Autodesk Fusion 360 part; units mm, degrees
(part 7 of 11)
  arc A26 (6.6572, -81.7997) -> (6.7986, -81.4582) centre (6.6572, -81.5997) ccw
  line L277 (19.9198, -134.2989) -> (19.8859, -134.2627)
  line L278 (4.42, -81.7997) -> (6.6572, -81.7997)
  line L279 (4.62, -81.9997) -> (6.6572, -81.9997)
  line L280 (20.0926, -134.6222) -> (20.0773, -134.5717)
  line L281 (19.9148, -134.7519) -> (19.9083, -134.7127)
  line L282 (4.42, -81.7997) -> (6.6572, -81.7997)
  arc A27 (6.6572, -81.7997) -> (6.7986, -81.4582) centre (6.6572, -81.5997) ccw
  line L283 (20.1046, -134.6736) -> (20.0926, -134.6222)
  line L284 (1.92, -84.6997) -> (3.2765, -84.6997)
  arc A28 (6.6572, -81.9997) -> (6.94, -81.3168) centre (6.6572, -81.5997) ccw
  line L285 (20.12, -134.8278) -> (20.1184, -134.7783)
  line L286 (4.42, -83.439) -> (4.42, -81.7997)
  line L287 (19.8993, -134.674) -> (19.8878, -134.636)
  line L288 (1.72, -84.4997) -> (3.3593, -84.4997)
  line L289 (20.012, -134.4275) -> (19.9841, -134.3827)
  line L290 (4.42, -83.439) -> (4.42, -81.7997)
  line L291 (19.9083, -134.7127) -> (19.8993, -134.674)
  line L292 (1.72, -84.4997) -> (3.3593, -84.4997)
  line L293 (-3, -220) -> (20, -220)
  line L294 (19.9148, -134.7519) -> (19.9083, -134.7127)
  line L295 (19.9841, -134.3827) -> (19.9533, -134.3397)
  line L296 (19.8878, -134.636) -> (19.8738, -134.5988)
  line L297 (-0.08, -85.0997) -> (-0.0787, -85.2079)
  line L298 (20.0587, -134.5222) -> (20.0369, -134.4741)
  line L299 (-0.28, -81.4997) -> (-0.28, -85.1009)
  line L300 (19.92, -134.8311) -> (19.9187, -134.7914)
  line L301 (-0.08, -85.0997) -> (-0.0787, -85.2079)
  line L302 (19.9187, -134.7914) -> (19.9148, -134.7519)
  line L303 (19.8387, -134.5276) -> (19.8177, -134.4938)
  line L304 (-0.28, -85.1009) -> (-0.2786, -85.2189)
  line L305 (-0.0787, -85.2079) -> (-0.0748, -85.2474)
  line L306 (-0.2786, -85.2189) -> (-0.2732, -85.2736)
  line L307 (20.1132, -134.7258) -> (20.1046, -134.6736)
  line L308 (20.0773, -134.5717) -> (20.0587, -134.5222)
  line L309 (19.8993, -134.674) -> (19.8878, -134.636)
  line L310 (19.9533, -134.3397) -> (19.9198, -134.2989)
  line L311 (20.1184, -134.7783) -> (20.1132, -134.7258)
  line L312 (18.12, -57.2997) -> (18.12, -62.6997)
  line L313 (-0.0787, -85.2079) -> (-0.0748, -85.2474)
  line L314 (-0.0748, -85.2474) -> (-0.0683, -85.2866)
  line L315 (19.8574, -134.5626) -> (19.8387, -134.5276)
  line L316 (-0.08, -81.4997) -> (-0.08, -85.0997)
  line L317 (-0.0683, -85.2866) -> (-0.0593, -85.3253)
  line L318 (19.7946, -134.4616) -> (19.7694, -134.4308)
  line L319 (7.0807, -86.0997) -> (4.42, -83.439)
  line L320 (3.3593, -84.4997) -> (6.02, -87.1603)
  line L321 (19.7946, -134.4616) -> (19.7694, -134.4308)
  line L322 (-0.2732, -85.2736) -> (-0.2646, -85.3257)
  line L323 (1.72, -86.7368) -> (1.72, -84.4997)
  line L324 (-0.08, -81.4997) -> (-0.08, -85.0997)
  line L325 (19.9083, -134.7127) -> (19.8993, -134.674)
  line L326 (19.8177, -134.4938) -> (19.7946, -134.4616)
  line L327 (19.8177, -134.4938) -> (19.7946, -134.4616)
  line L328 (-0.0748, -85.2474) -> (-0.0683, -85.2866)
  line L329 (19.9187, -134.7914) -> (19.9148, -134.7519)
  line L330 (7.1635, -85.8997) -> (4.62, -83.3562)
  line L331 (19.8738, -134.5988) -> (19.8574, -134.5626)
  line L332 (1.92, -86.7368) -> (1.92, -84.6997)
  line L333 (7.0807, -86.0997) -> (4.42, -83.439)
  line L334 (19.92, -134.8311) -> (19.9187, -134.7914)
  line L335 (19.8878, -134.636) -> (19.8738, -134.5988)
  line L336 (20.0369, -134.4741) -> (20.012, -134.4275)
  line L337 (-0.0683, -85.2866) -> (-0.0593, -85.3253)
  line L338 (19.8387, -134.5276) -> (19.8177, -134.4938)
  line L339 (1.72, -86.7368) -> (1.72, -84.4997)
  line L340 (19.8574, -134.5626) -> (19.8387, -134.5276)
  line L341 (3.3593, -84.4997) -> (6.02, -87.1603)
  line L342 (3.2765, -84.6997) -> (5.82, -87.2432)
  line L343 (9.7959, -85.8997) -> (7.1635, -85.8997)
  circle A29 centre (9.92, -89.9997) radius 2.1
  arc A30 (18.6028, -132.9797) -> (17.92, -133.2625) centre (18.32, -133.2625) ccw
  line L344 (19.8993, -154.674) -> (19.8878, -154.636)
  line L345 (19.8574, -154.5626) -> (19.8387, -154.5276)
  line L346 (20.1046, -154.6736) -> (20.0926, -154.6222)
  line L347 (19.7946, -154.4616) -> (19.7694, -154.4308)
  line L348 (20.0369, -154.4741) -> (20.012, -154.4275)
  line L349 (19.9083, -154.7127) -> (19.8993, -154.674)
  line L350 (19.8738, -154.5988) -> (19.8574, -154.5626)
  line L351 (19.7694, -154.4308) -> (19.7422, -154.4019)
  line L352 (20.0773, -154.5717) -> (20.0587, -154.5222)
  line L353 (7.0807, -6.0997) -> (4.42, -3.439)
  line L354 (1.72, -4.4997) -> (3.3593, -4.4997)
  line L355 (19.92, -1.4997) -> (19.92, -0.4997)
  line L356 (-0.0787, -5.2079) -> (-0.0748, -5.2474)
  line L357 (18.42, 0.0003) -> (14.7514, 0.0003)
  arc A31 (19.92, -0.4997) -> (19.42, 0.0003) centre (19.42, -0.4997) ccw
  line L358 (3.3593, -4.4997) -> (6.02, -7.1603)
  line L359 (19.92, -1.4997) -> (19.92, -0.4997)
  line L360 (19.7946, -14.4616) -> (19.7694, -14.4308)
  line L361 (-0.0459, -5.7366) -> (1.2372, -7.0197)
  line L362 (9.713, -26.0997) -> (7.0807, -26.0997)
  line L363 (9.713, -26.0997) -> (7.0807, -26.0997)
  line L364 (19.9841, -14.3827) -> (19.9533, -14.3397)
  line L365 (19.9083, -45.2866) -> (19.9148, -45.2474)
  line L366 (-0.0683, -5.2866) -> (-0.0593, -5.3253)
  line L367 (10.127, -13.8997) -> (12.7593, -13.8997)
  line L368 (19.9533, -14.3397) -> (19.9198, -14.2989)
  line L369 (19.7694, -14.4308) -> (19.7422, -14.4019)
  line L370 (20.12, -1.4997) -> (20.12, -0.4997)
  line L371 (19.8177, -14.4938) -> (19.7946, -14.4616)
  line L372 (7.0807, -6.0997) -> (4.42, -3.439)
  line L373 (19.92, -14.8997) -> (19.9187, -14.7914)
  line L374 (19.8993, -14.674) -> (19.8878, -14.636)
  line L375 (4.62, -1.9997) -> (6.6572, -1.9997)
  arc A32 (1.2372, -27.0197) -> (1.92, -26.7368) centre (1.52, -26.7368) ccw
  line L376 (19.9148, -14.7519) -> (19.9083, -14.7127)
  line L377 (19.42, 0.2003) -> (18.42, 0.2003)
  line L378 (0.0978, -5.5975) -> (1.3786, -6.8782)
  line L379 (18.42, 0.2003) -> (14.7482, 0.2003)
  line L380 (1.72, -4.4997) -> (3.3593, -4.4997)
  line L381 (19.42, 0.0003) -> (18.42, 0.0003)
  line L382 (7.1635, -5.8997) -> (4.62, -3.3562)
  line L383 (-0.0748, -5.2474) -> (-0.0683, -5.2866)
  line L384 (19.7946, -45.5378) -> (19.8177, -45.5055)
  line L385 (19.8738, -45.4005) -> (19.8878, -45.3633)
  line L386 (9.92, -26.3066) -> (9.713, -26.0997)
  line L387 (9.7959, -14.0997) -> (9.92, -13.9755)
  arc A33 (19.92, -0.4997) -> (19.42, 0.0003) centre (19.42, -0.4997) ccw
  line L388 (3.2765, -4.6997) -> (5.82, -7.2432)
  line L389 (19.42, 0.0003) -> (18.42, 0.0003)
  line L390 (19.8177, -14.4938) -> (19.7946, -14.4616)
  line L391 (12.7593, -26.0997) -> (10.127, -26.0997)
  line L392 (7.0807, -13.8997) -> (9.713, -13.8997)
  line L393 (1.92, -6.7368) -> (1.92, -4.6997)
  line L394 (-0.28, -5.1009) -> (-0.2786, -5.2189)
  line L395 (20.1046, -14.6736) -> (20.0926, -14.6222)
  line L396 (19.8387, -14.5276) -> (19.8177, -14.4938)
  line L397 (20.0773, -14.5717) -> (20.0587, -14.5222)
  arc A34 (6.6572, -1.7997) -> (6.7986, -1.4582) centre (6.6572, -1.5997) ccw
  arc A35 (20.12, -0.4997) -> (19.42, 0.2003) centre (19.42, -0.4997) ccw
  line L398 (1.72, -6.7368) -> (1.72, -4.4997)
  line L399 (10.127, -13.8997) -> (12.7593, -13.8997)
  line L400 (3.3593, -4.4997) -> (6.02, -7.1603)
  line L401 (3.7635, -162.4997) -> (1.92, -162.4997)
  line L402 (1.72, -6.7368) -> (1.72, -4.4997)
  line L403 (18.42, 0.0003) -> (14.7514, 0.0003)
  line L404 (19.8878, -14.636) -> (19.8738, -14.5988)
  arc A36 (1.2372, -167.0197) -> (1.92, -166.7368) centre (1.52, -166.7368) ccw
  line L405 (9.92, -13.6927) -> (10.127, -13.8997)
  line L406 (19.7946, -14.4616) -> (19.7694, -14.4308)
  line L407 (19.9083, -14.7127) -> (19.8993, -14.674)
  line L408 (0.0978, -5.5975) -> (1.3786, -6.8782)
  line L409 (19.92, -14.8997) -> (19.9187, -14.7914)
  line L410 (19.7694, -14.4308) -> (19.7422, -14.4019)
  line L411 (5.4921, 0.0923) -> (5.4455, 0.1172)
  line L412 (0.0978, -25.5975) -> (1.3786, -26.8782)
  line L413 (-0.0593, -25.3253) -> (-0.0478, -25.3633)
  line L414 (19.8574, -14.5626) -> (19.8387, -14.5276)
  line L415 (19.9187, -14.7914) -> (19.9148, -14.7519)
  line L416 (6.7986, -1.4582) -> (5.5178, -0.1775)
  arc A37 (6.6572, -1.7997) -> (6.7986, -1.4582) centre (6.6572, -1.5997) ccw
  line L417 (4.42, -1.7997) -> (6.6572, -1.7997)
  line L418 (20.012, -14.4275) -> (19.9841, -14.3827)
  line L419 (-0.1969, -25.5252) -> (-0.172, -25.5718)
  line L420 (14.6722, -0.0049) -> (14.633, -0.0113)
  line L421 (14.5943, -0.0203) -> (14.5563, -0.0319)
  line L422 (14.3945, 0.1172) -> (14.3479, 0.0923)
  line L423 (5.4581, -0.1251) -> (5.4258, -0.102)
  line L424 (6.7986, -1.4582) -> (5.5178, -0.1775)
  line L425 (19.8878, -14.636) -> (19.8738, -14.5988)
  line L426 (19.8738, -14.5988) -> (19.8574, -14.5626)
  line L427 (19.9083, -14.7127) -> (19.8993, -14.674)
  line L428 (19.9187, -14.7914) -> (19.9148, -14.7519)
  line L429 (5.3974, 0.139) -> (5.348, 0.1576)
  line L430 (20.0587, -14.5222) -> (20.0369, -14.4741)
  arc A38 (1.3786, -26.8782) -> (1.72, -26.7368) centre (1.52, -26.7368) ccw
  line L431 (14.6987, 0.1987) -> (14.6461, 0.1935)
  line L432 (20.1132, -14.7258) -> (20.1046, -14.6736)
  line L433 (14.4142, -0.102) -> (14.3819, -0.1251)
  line L434 (20.12, -14.8985) -> (20.1186, -14.7804)
  line L435 (-0.2732, -25.2736) -> (-0.2646, -25.3257)
  arc A39 (1.3786, -26.8782) -> (1.72, -26.7368) centre (1.52, -26.7368) ccw
  line L436 (14.3512, -0.1503) -> (14.3222, -0.1775)
  line L437 (14.4479, -0.081) -> (14.4142, -0.102)
  line L438 (14.633, -0.0113) -> (14.5943, -0.0203)
  line L439 (5.537, 0.0644) -> (5.4921, 0.0923)
  line L440 (14.594, 0.1849) -> (14.5425, 0.1729)
  line L441 (19.8993, -14.674) -> (19.8878, -14.636)
  line L442 (-0.2786, -25.2189) -> (-0.2732, -25.2736)
  line L443 (5.4258, -0.102) -> (5.3921, -0.081)
  arc A40 (6.6572, -1.9997) -> (6.94, -1.3168) centre (6.6572, -1.5997) ccw
  line L444 (-0.0338, -25.4005) -> (-0.0174, -25.4367)
  line L445 (5.2837, -0.0319) -> (5.2457, -0.0203)
  line L446 (14.3512, -0.1503) -> (14.3222, -0.1775)
  line L447 (5.2457, -0.0203) -> (5.207, -0.0113)
  line L448 (5.2457, -0.0203) -> (5.207, -0.0113)
  line L449 (-0.28, -25.1009) -> (-0.2786, -25.2189)
  line L450 (19.8574, -14.5626) -> (19.8387, -14.5276)
  line L451 (-0.1133, -25.6596) -> (-0.0798, -25.7004)
  line L452 (19.8738, -14.5988) -> (19.8574, -14.5626)
  line L453 (19.8387, -14.5276) -> (19.8177, -14.4938)
  line L454 (0.0978, -25.5975) -> (1.3786, -26.8782)
  line L455 (4.42, -1.7997) -> (6.6572, -1.7997)
  line L456 (19.9198, -14.2989) -> (19.8859, -14.2627)
  line L457 (20.1186, -14.7804) -> (20.1132, -14.7258)
  line L458 (20.0369, -14.4741) -> (20.012, -14.4275)
  arc A41 (18.6028, -12.9797) -> (17.92, -13.2625) centre (18.32, -13.2625) ccw
  line L459 (19.9148, -14.7519) -> (19.9083, -14.7127)
  line L460 (20.0926, -14.6222) -> (20.0773, -14.5717)
  line L461 (-0.0748, -25.2474) -> (-0.0683, -25.2866)
  line L462 (5.2975, 0.1729) -> (5.246, 0.1849)
  line L463 (-0.0748, -25.2474) -> (-0.0683, -25.2866)
  arc A42 (18.4614, -13.1211) -> (18.12, -13.2625) centre (18.32, -13.2625) ccw
  line L464 (-0.0787, -25.2079) -> (-0.0748, -25.2474)
  arc A43 (18.4614, -13.1211) -> (18.12, -13.2625) centre (18.32, -13.2625) ccw
  line L465 (-0.0338, -25.4005) -> (-0.0174, -25.4367)
  line L466 (14.3819, -0.1251) -> (14.3512, -0.1503)
  line L467 (18.12, -13.2625) -> (18.12, -15.4997)
  line L468 (14.633, -0.0113) -> (14.5943, -0.0203)
  line L469 (5.2837, -0.0319) -> (5.2457, -0.0203)
  line L470 (-0.0174, -25.4367) -> (0.0013, -25.4717)
  line L471 (17.92, -13.2625) -> (17.92, -15.2997)
  line L472 (14.6461, 0.1935) -> (14.594, 0.1849)
  line L473 (-0.0787, -25.2079) -> (-0.0748, -25.2474)
  line L474 (5.4258, -0.102) -> (5.3921, -0.081)
  line L475 (5.246, 0.1849) -> (5.1939, 0.1935)
  line L476 (0.0223, -25.5055) -> (0.0454, -25.5378)
  line L477 (14.3479, 0.0923) -> (14.303, 0.0644)
  line L478 (-0.1441, -25.6166) -> (-0.1133, -25.6596)
  line L479 (6.02, -12.839) -> (3.3593, -15.4997)
  line L480 (5.348, 0.1576) -> (5.2975, 0.1729)
  line L481 (16.4807, -15.4997) -> (13.82, -12.839)
  line L482 (0.0013, -25.4717) -> (0.0223, -25.5055)
  line L483 (14.4479, -0.081) -> (14.4142, -0.102)
  line L484 (5.1283, -0.001) -> (5.0886, 0.0003)
  line L485 (-0.08, -25.0997) -> (-0.0787, -25.2079)
  line L486 (-0.0174, -25.4367) -> (0.0013, -25.4717)
  line L487 (19.92, -25.0997) -> (19.92, -14.8997)
  line L488 (5.1283, -0.001) -> (5.0886, 0.0003)
  line L489 (-0.08, -25.0997) -> (-0.0787, -25.2079)
  line L490 (5.1413, 0.1987) -> (5.0918, 0.2003)
  line L491 (-0.2526, -25.3771) -> (-0.2373, -25.4277)
  line L492 (18.12, -13.2625) -> (18.12, -15.4997)
  line L493 (5.207, -0.0113) -> (5.1678, -0.0049)
  line L494 (5.3921, -0.081) -> (5.357, -0.0623)
  line L495 (14.483, -0.0623) -> (14.4479, -0.081)
  line L496 (19.7422, -14.4019) -> (18.4614, -13.1211)
  line L497 (16.5635, -15.2997) -> (14.02, -12.7562)
  line L498 (5.357, -0.0623) -> (5.3209, -0.0459)
  line L499 (14.5191, -0.0459) -> (14.483, -0.0623)
  line L500 (17.92, -15.2997) -> (16.5635, -15.2997)
  line L501 (5.3209, -0.0459) -> (5.2837, -0.0319)
  line L502 (-0.0683, -25.2866) -> (-0.0593, -25.3253)
  line L503 (0.0454, -25.5378) -> (0.0706, -25.5685)
  line L504 (-0.0683, -25.2866) -> (-0.0593, -25.3253)
  line L505 (-0.172, -25.5718) -> (-0.1441, -25.6166)
  line L506 (14.7117, -0.001) -> (14.6722, -0.0049)
  line L507 (0.0454, -25.5378) -> (0.0706, -25.5685)
  line L508 (18.12, -15.4997) -> (16.4807, -15.4997)
  line L509 (5.5799, 0.0337) -> (5.537, 0.0644)
  line L510 (19.7422, -14.4019) -> (18.4614, -13.1211)
  line L511 (0.0013, -25.4717) -> (0.0223, -25.5055)
  line L512 (5.1678, -0.0049) -> (5.1283, -0.001)
  line L513 (14.5563, -0.0319) -> (14.5191, -0.0459)
  line L514 (5.6207, 0.0001) -> (5.5799, 0.0337)
  line L515 (19.8859, -14.2627) -> (18.6028, -12.9797)
  line L516 (-0.2373, -25.4277) -> (-0.2187, -25.4771)
  line L517 (-0.0798, -25.7004) -> (-0.0459, -25.7366)
  line L518 (16.4807, -15.4997) -> (13.82, -12.839)
  line L519 (-0.0593, -25.3253) -> (-0.0478, -25.3633)
  line L520 (5.6569, -0.0337) -> (5.6207, 0.0001)
  line L521 (18.12, -15.4997) -> (16.4807, -15.4997)
  line L522 (5.1678, -0.0049) -> (5.1283, -0.001)
  line L523 (-0.0478, -25.3633) -> (-0.0338, -25.4005)
  line L524 (5.4888, -0.1503) -> (5.4581, -0.1251)
  line L525 (20.12, -25.1009) -> (20.12, -14.8985)
  line L526 (14.303, 0.0644) -> (14.2601, 0.0337)
  line L527 (-0.0478, -25.3633) -> (-0.0338, -25.4005)
  line L528 (5.4888, -0.1503) -> (5.4581, -0.1251)
  line L529 (14.5425, 0.1729) -> (14.492, 0.1576)
  line L530 (19.92, -25.0997) -> (19.92, -14.8997)
  line L531 (4.42, -3.439) -> (4.42, -1.7997)
  line L532 (3.3593, -24.4997) -> (6.02, -27.1603)
  line L533 (-0.0459, -25.7366) -> (1.2372, -27.0197)
  line L534 (14.5191, -0.0459) -> (14.483, -0.0623)
  line L535 (-0.08, -0.4997) -> (-0.08, -1.4997)
  line L536 (14.2601, 0.0337) -> (14.2193, 0.0001)
  line L537 (0.0706, -25.5685) -> (0.0978, -25.5975)
  line L538 (14.492, 0.1576) -> (14.4426, 0.139)
  line L539 (6.94, -1.3168) -> (5.6569, -0.0337)
  line L540 (1.72, -17.2997) -> (3.6807, -17.2997)
  line L541 (5.4581, -0.1251) -> (5.4258, -0.102)
  line L542 (19.92, -5.1682) -> (19.92, -1.4997)
  line L543 (7.0807, -46.0997) -> (3.6807, -42.6997)
  line L544 (3.6807, -22.6997) -> (1.72, -22.6997)
  line L545 (5.1939, 0.1935) -> (5.1413, 0.1987)
  line L546 (14.483, -0.0623) -> (14.4479, -0.081)
  line L547 (5.3209, -0.0459) -> (5.2837, -0.0319)
  line L548 (5.207, -0.0113) -> (5.1678, -0.0049)
  line L549 (5.5178, -0.1775) -> (5.4888, -0.1503)
  line L550 (13.82, -7.1603) -> (16.4807, -4.4997)
  line L551 (14.5563, -0.0319) -> (14.5191, -0.0459)
  line L552 (-0.2187, -25.4771) -> (-0.1969, -25.5252)
  line L553 (1.92, -17.4997) -> (3.7635, -17.4997)
  line L554 (0.0223, -25.5055) -> (0.0454, -25.5378)
  line L555 (1.72, -22.6997) -> (1.72, -17.2997)
  line L556 (7.0807, -26.0997) -> (3.6807, -22.6997)
  line L557 (14.6722, -0.0049) -> (14.633, -0.0113)
  line L558 (14.5943, -0.0203) -> (14.5563, -0.0319)
  line L559 (13.82, -192.839) -> (13.82, -190.1995)
  line L560 (15.42, -3.439) -> (12.7593, -6.0997)
  line L561 (5.4455, 0.1172) -> (5.3974, 0.139)
  line L562 (19.92, -45.0997) -> (19.92, -34.8997)
  line L563 (1.72, -22.6997) -> (1.72, -17.2997)
  line L564 (5.3921, -0.081) -> (5.357, -0.0623)
  line L565 (3.7635, -22.4997) -> (1.92, -22.4997)
  line L566 (3.2765, -24.6997) -> (5.82, -27.2432)
  line L567 (14.7514, 0.0003) -> (14.7117, -0.001)
  line L568 (5.5178, -0.1775) -> (5.4888, -0.1503)
  line L569 (16.1593, -42.6997) -> (12.7593, -46.0997)
  line L570 (1.92, -24.6997) -> (3.2765, -24.6997)
  line L571 (13.1828, -1.7997) -> (15.42, -1.7997)
  line L572 (3.6807, -22.6997) -> (1.72, -22.6997)
  arc A44 (0.42, 0.2003) -> (-0.28, -0.4997) centre (0.42, -0.4997) ccw
  line L573 (14.3819, -0.1251) -> (14.3512, -0.1503)
  line L574 (14.4142, -0.102) -> (14.3819, -0.1251)
  line L575 (1.72, -24.4997) -> (3.3593, -24.4997)
  line L576 (20.12, -5.1715) -> (20.12, -1.4997)
  line L577 (13.82, -192.839) -> (13.82, -190.1995)
  arc A45 (0.42, 0.0003) -> (-0.08, -0.4997) centre (0.42, -0.4997) ccw
  line L578 (1.72, -24.4997) -> (3.3593, -24.4997)
  line L579 (15.42, -1.7997) -> (15.42, -3.439)
  line L580 (14.7117, -0.001) -> (14.6722, -0.0049)
  line L581 (14.4426, 0.139) -> (14.3945, 0.1172)
  line L582 (5.357, -0.0623) -> (5.3209, -0.0459)
  line L583 (14.7482, 0.2003) -> (14.6987, 0.1987)
  line L584 (0.0706, -25.5685) -> (0.0978, -25.5975)
  line L585 (14.7514, 0.0003) -> (14.7117, -0.001)
  line L586 (7.1635, -25.8997) -> (3.7635, -22.4997)
  line L587 (-0.2646, -25.3257) -> (-0.2526, -25.3771)
  line L588 (1.92, -22.4997) -> (1.92, -17.4997)
  line L589 (15.22, -1.9997) -> (15.22, -3.3562)
  line L590 (19.92, -5.1682) -> (19.92, -1.4997)
  line L591 (1.72, -17.2997) -> (3.6807, -17.2997)
  line L592 (1.42, 0.0003) -> (0.42, 0.0003)
  line L593 (1.72, -26.7368) -> (1.72, -24.4997)
  line L594 (19.8993, -194.674) -> (19.8878, -194.636)
  line L595 (19.9187, -194.7914) -> (19.9148, -194.7519)
  line L596 (12.7593, -6.0997) -> (10.127, -6.0997)
  line L597 (20.12, -194.8985) -> (20.1186, -194.7804)
  line L598 (1.72, -15.4997) -> (1.72, -13.2625)
  line L599 (13.6201, -9.9997) -> (13.82, -9.7998)
  line L600 (14.02, -10.1167) -> (13.903, -9.9997)
  line L601 (5.0886, 0.0003) -> (1.42, 0.0003)
  line L602 (13.903, -9.9997) -> (14.02, -9.8826)
  line L603 (19.9083, -194.7127) -> (19.8993, -194.674)
  line L604 (19.9148, -34.7519) -> (19.9083, -34.7127)
  line L605 (1.72, -26.7368) -> (1.72, -24.4997)
  arc A46 (1.92, -13.2625) -> (1.2372, -12.9797) centre (1.52, -13.2625) ccw
  line L606 (19.8177, -194.4938) -> (19.7946, -194.4616)
  line L607 (0.0706, -14.4308) -> (0.0454, -14.4616)
  line L608 (19.9187, -34.7914) -> (19.9148, -34.7519)
  line L609 (15.42, -1.7997) -> (15.42, -3.439)
  line L610 (5.0918, 0.2003) -> (1.42, 0.2003)
  line L611 (3.3593, -15.4997) -> (1.72, -15.4997)
  line L612 (7.1635, -45.8997) -> (3.7635, -42.4997)
  line L613 (19.7946, -194.4616) -> (19.7694, -194.4308)
  arc A47 (1.72, -13.2625) -> (1.3786, -13.1211) centre (1.52, -13.2625) ccw
  line L614 (1.3786, -13.1211) -> (0.0978, -14.4019)
  line L615 (19.9841, -194.3827) -> (19.9533, -194.3397)
  line L616 (1.42, 0.2003) -> (0.42, 0.2003)
  line L617 (3.3593, -15.4997) -> (1.72, -15.4997)
  line L618 (19.8177, -194.4938) -> (19.7946, -194.4616)
  line L619 (20.1186, -194.7804) -> (20.1132, -194.7258)
  line L620 (19.8387, -194.5276) -> (19.8177, -194.4938)
  line L621 (19.9148, -194.7519) -> (19.9083, -194.7127)
  arc A48 (13.0414, -1.4582) -> (13.1828, -1.7997) centre (13.1828, -1.5997) ccw
  arc A49 (12.9, -1.3168) -> (13.1828, -1.9997) centre (13.1828, -1.5997) ccw
  line L622 (12.7593, -6.0997) -> (10.127, -6.0997)
  line L623 (1.42, 0.0003) -> (0.42, 0.0003)
  arc A50 (0.42, 0.0003) -> (-0.08, -0.4997) centre (0.42, -0.4997) ccw
  line L624 (1.3786, -13.1211) -> (0.0978, -14.4019)
  line L625 (19.8738, -194.5988) -> (19.8574, -194.5626)
  line L626 (17.92, -37.4997) -> (17.92, -42.4997)
  line L627 (5.0886, 0.0003) -> (1.42, 0.0003)
  circle A51 centre (9.92, -9.9997) radius 2.1
  line L628 (19.9198, -194.2989) -> (19.8859, -194.2627)
  line L629 (19.8387, -194.5276) -> (19.8177, -194.4938)
  line L630 (20.0926, -194.6222) -> (20.0773, -194.5717)
  line L631 (-0.08, -0.4997) -> (-0.08, -1.4997)
  line L632 (-0.28, -0.4997) -> (-0.28, -1.4997)
  line L633 (-0.28, -1.4997) -> (-0.28, -5.1009)
  arc A52 (1.72, -13.2625) -> (1.3786, -13.1211) centre (1.52, -13.2625) ccw
  line L634 (1.92, -15.2997) -> (1.92, -13.2625)
  line L635 (9.9208, -6.0223) -> (9.7981, -5.8997)
  line L636 (1.92, -26.7368) -> (1.92, -24.6997)
  line L637 (3.2765, -15.2997) -> (1.92, -15.2997)
  line L638 (1.72, -15.4997) -> (1.72, -13.2625)
  line L639 (13.82, -9.7998) -> (13.82, -7.1603)
  line L640 (10.127, -6.0997) -> (9.92, -6.3044)
  line L641 (19.7694, -194.4308) -> (19.7422, -194.4019)
  line L642 (12.6765, -5.8997) -> (10.0448, -5.8997)
  line L643 (17.92, -42.4997) -> (16.0765, -42.4997)
  circle A53 centre (9.92, -9.9997) radius 2.1
  line L644 (16.0765, -37.4997) -> (17.92, -37.4997)
  line L645 (10.0448, -5.8997) -> (9.9208, -6.0223)
  line L646 (-0.172, -14.4275) -> (-0.1969, -14.4741)
  line L647 (14.1831, -0.0337) -> (12.9, -1.3168)
  line L648 (-0.1133, -14.3397) -> (-0.1441, -14.3827)
  line L649 (16.1593, -37.2997) -> (18.12, -37.2997)
  line L650 (14.02, -9.8826) -> (14.02, -7.2432)
  line L651 (9.92, -6.3044) -> (9.7152, -6.0997)
  line L652 (-0.2187, -14.5222) -> (-0.2373, -14.5717)
  line L653 (-0.0174, -14.5626) -> (-0.0338, -14.5988)
  line L654 (6.02, -207.1603) -> (6.02, -209.7998)
  line L655 (19.7946, -194.4616) -> (19.7694, -194.4308)
  line L656 (-0.0798, -14.2989) -> (-0.1133, -14.3397)
  line L657 (20.0369, -194.4741) -> (20.012, -194.4275)
  line L658 (-0.0338, -14.5988) -> (-0.0478, -14.636)
  line L659 (9.92, -6.3044) -> (9.7152, -6.0997)
  line L660 (-0.2526, -14.6222) -> (-0.2646, -14.6736)
  line L661 (20.0587, -194.5222) -> (20.0369, -194.4741)
  line L662 (20.1046, -34.6736) -> (20.0926, -34.6222)
  line L663 (10.127, -6.0997) -> (9.92, -6.3044)
  line L664 (18.12, -42.6997) -> (16.1593, -42.6997)
  line L665 (19.9083, -34.7127) -> (19.8993, -34.674)
  line L666 (13.82, -10.1995) -> (13.6201, -9.9997)
  line L667 (-0.1969, -14.4741) -> (-0.2187, -14.5222)
  line L668 (19.8574, -34.5626) -> (19.8387, -34.5276)
  line L669 (0.0454, -14.4616) -> (0.0223, -14.4938)
  line L670 (20.1132, -194.7258) -> (20.1046, -194.6736)
  line L671 (20.12, -34.8985) -> (20.1186, -34.7804)
  line L672 (19.9148, -194.7519) -> (19.9083, -194.7127)
  line L673 (19.8738, -194.5988) -> (19.8574, -194.5626)
  line L674 (19.8878, -194.636) -> (19.8738, -194.5988)
  line L675 (20.0926, -34.6222) -> (20.0773, -34.5717)
  line L676 (13.6201, -9.9997) -> (13.82, -9.7998)
  line L677 (-0.0748, -14.7519) -> (-0.0787, -14.7914)
  line L678 (19.9083, -194.7127) -> (19.8993, -194.674)
  line L679 (18.12, -37.2997) -> (18.12, -42.6997)
  line L680 (6.02, -12.839) -> (3.3593, -15.4997)
  line L681 (19.9187, -194.7914) -> (19.9148, -194.7519)
  line L682 (-0.0683, -14.7127) -> (-0.0748, -14.7519)
  line L683 (19.9533, -194.3397) -> (19.9198, -194.2989)
  line L684 (20.0926, -45.3771) -> (20.1046, -45.3257)
  line L685 (-0.0787, -14.7914) -> (-0.08, -14.8997)
  line L686 (16.1593, -37.2997) -> (18.12, -37.2997)
  line L687 (13.82, -9.7998) -> (13.82, -7.1603)
  line L688 (-0.0478, -14.636) -> (-0.0593, -14.674)
  line L689 (18.12, -35.4997) -> (16.4807, -35.4997)
  line L690 (19.8878, -34.636) -> (19.8738, -34.5988)
  line L691 (-0.2786, -14.7804) -> (-0.28, -14.8985)
  line L692 (19.8993, -34.674) -> (19.8878, -34.636)
  line L693 (20.0773, -34.5717) -> (20.0587, -34.5222)
  line L694 (19.8878, -194.636) -> (19.8738, -194.5988)
  line L695 (20.012, -194.4275) -> (19.9841, -194.3827)
  line L696 (0.0706, -14.4308) -> (0.0454, -14.4616)
  line L697 (18.12, -37.2997) -> (18.12, -42.6997)
  line L698 (19.8993, -194.674) -> (19.8878, -194.636)
  arc A54 (13.0414, -1.4582) -> (13.1828, -1.7997) centre (13.1828, -1.5997) ccw
  line L699 (14.2193, 0.0001) -> (14.1831, -0.0337)
  line L700 (19.8993, -34.674) -> (19.8878, -34.636)
  line L701 (-0.0338, -14.5988) -> (-0.0478, -14.636)
  line L702 (17.92, -35.2997) -> (16.5635, -35.2997)
  line L703 (19.92, -34.8997) -> (19.9187, -34.7914)
  line L704 (19.8574, -194.5626) -> (19.8387, -194.5276)
  line L705 (19.92, -194.8997) -> (19.9187, -194.7914)
  line L706 (-0.2373, -14.5717) -> (-0.2526, -14.6222)
  line L707 (19.8878, -34.636) -> (19.8738, -34.5988)
  line L708 (13.82, -10.1995) -> (13.6201, -9.9997)
  line L709 (13.82, -209.7998) -> (13.82, -207.1603)
  line L710 (20.0773, -194.5717) -> (20.0587, -194.5222)
  line L711 (0.0223, -14.4938) -> (0.0013, -14.5276)
  line L712 (19.8574, -194.5626) -> (19.8387, -194.5276)
  line L713 (20.1186, -34.7804) -> (20.1132, -34.7258)
  line L714 (19.8878, -45.3633) -> (19.8993, -45.3253)
  line L715 (19.92, -185.0997) -> (19.92, -174.8997)
  line L716 (19.7946, -45.5378) -> (19.8177, -45.5055)
  line L717 (-0.0683, -14.7127) -> (-0.0748, -14.7519)
  line L718 (0.0013, -14.5276) -> (-0.0174, -14.5626)
  line L719 (-0.0787, -14.7914) -> (-0.08, -14.8997)
  line L720 (19.8738, -34.5988) -> (19.8574, -34.5626)
  line L721 (9.7959, -45.8997) -> (7.1635, -45.8997)
  line L722 (0.0978, -14.4019) -> (0.0706, -14.4308)
  line L723 (19.9148, -34.7519) -> (19.9083, -34.7127)
  line L724 (20.1132, -34.7258) -> (20.1046, -34.6736)
  line L725 (7.0807, -33.8997) -> (9.713, -33.8997)
  line L726 (19.8177, -45.5055) -> (19.8387, -45.4717)
  line L727 (-0.0478, -14.636) -> (-0.0593, -14.674)
  line L728 (19.9083, -34.7127) -> (19.8993, -34.674)
  line L729 (19.9841, -45.6166) -> (20.012, -45.5718)
  line L730 (19.8993, -45.3253) -> (19.9083, -45.2866)
  line L731 (19.7694, -194.4308) -> (19.7422, -194.4019)
  line L732 (-0.0174, -14.5626) -> (-0.0338, -14.5988)
  line L733 (3.6807, -17.2997) -> (7.0807, -13.8997)
  line L734 (19.92, -194.8997) -> (19.9187, -194.7914)
  line L735 (5.82, -12.7562) -> (3.2765, -15.2997)
  line L736 (19.8738, -45.4005) -> (19.8878, -45.3633)
  line L737 (-0.0593, -14.674) -> (-0.0683, -14.7127)
  line L738 (0.0013, -14.5276) -> (-0.0174, -14.5626)
  line L739 (18.12, -42.6997) -> (16.1593, -42.6997)
  line L740 (19.9148, -45.2474) -> (19.9187, -45.2079)
  line L741 (19.8859, -45.7366) -> (19.9198, -45.7004)
  line L742 (20.1046, -194.6736) -> (20.0926, -194.6222)
  line L743 (19.8574, -45.4367) -> (19.8738, -45.4005)
  line L744 (-0.2646, -14.6736) -> (-0.2732, -14.7258)
  line L745 (16.4807, -195.4997) -> (13.82, -192.839)
  line L746 (-0.0748, -14.7519) -> (-0.0787, -14.7914)
  line L747 (19.8738, -34.5988) -> (19.8574, -34.5626)
  line L748 (14.02, -209.8826) -> (14.02, -207.2432)
  line L749 (9.713, -46.0997) -> (7.0807, -46.0997)
  line L750 (19.7694, -45.5685) -> (19.7946, -45.5378)
  line L751 (-0.0593, -14.674) -> (-0.0683, -14.7127)
  line L752 (-0.1441, -14.3827) -> (-0.172, -14.4275)
  line L753 (0.0223, -14.4938) -> (0.0013, -14.5276)
  line L754 (18.12, -35.4997) -> (16.4807, -35.4997)
  line L755 (20.1046, -45.3257) -> (20.1132, -45.2736)
  line L756 (16.5635, -195.2997) -> (14.02, -192.7562)
  line L757 (9.713, -46.0997) -> (7.0807, -46.0997)
  line L758 (19.9187, -34.7914) -> (19.9148, -34.7519)
  line L759 (-0.2732, -14.7258) -> (-0.2786, -14.7804)
  line L760 (20.0773, -45.4277) -> (20.0926, -45.3771)
  line L761 (19.8574, -45.4367) -> (19.8738, -45.4005)
  line L762 (-0.0459, -14.2627) -> (-0.0798, -14.2989)
  line L763 (20.1132, -45.2736) -> (20.1186, -45.2189)
  line L764 (19.92, -34.8997) -> (19.9187, -34.7914)
  line L765 (19.8574, -34.5626) -> (19.8387, -34.5276)
  line L766 (16.4807, -195.4997) -> (13.82, -192.839)
  line L767 (17.92, -193.2625) -> (17.92, -195.2997)
  line L768 (7.0807, -53.8997) -> (9.713, -53.8997)
  line L769 (19.8993, -45.3253) -> (19.9083, -45.2866)
  line L770 (18.12, -195.4997) -> (16.4807, -195.4997)
  line L771 (7.1635, -34.0997) -> (9.7959, -34.0997)
  line L772 (0.0454, -14.4616) -> (0.0223, -14.4938)
  arc A55 (18.6028, -192.9797) -> (17.92, -193.2625) centre (18.32, -193.2625) ccw
  line L773 (-0.08, -174.8997) -> (-0.08, -185.0997)
  arc A56 (18.4614, -193.1211) -> (18.12, -193.2625) centre (18.32, -193.2625) ccw
  line L774 (3.6807, -17.2997) -> (7.0807, -13.8997)
  arc A57 (18.6028, -32.9797) -> (17.92, -33.2625) centre (18.32, -33.2625) ccw
  line L775 (3.3593, -24.4997) -> (6.02, -27.1603)
  line L776 (-0.08, -14.8997) -> (-0.08, -25.0997)
  line L777 (18.12, -193.2625) -> (18.12, -195.4997)
  line L778 (19.9533, -34.3397) -> (19.9198, -34.2989)
  line L779 (20.0369, -34.4741) -> (20.012, -34.4275)
  line L780 (3.7635, -17.4997) -> (7.1635, -14.0997)
  line L781 (3.7635, -177.4997) -> (7.1635, -174.0997)
  arc A58 (18.4614, -193.1211) -> (18.12, -193.2625) centre (18.32, -193.2625) ccw
  line L782 (7.0807, -53.8997) -> (9.713, -53.8997)
  line L783 (0.0978, -14.4019) -> (0.0706, -14.4308)
  line L784 (1.2372, -12.9797) -> (-0.0459, -14.2627)
  line L785 (18.12, -195.4997) -> (16.4807, -195.4997)
  line L786 (19.9083, -145.2866) -> (19.9148, -145.2474)
  line L787 (19.9148, -94.7519) -> (19.9083, -94.7127)
  line L788 (20.0773, -94.5717) -> (20.0587, -94.5222)
  line L789 (20.1132, -94.7258) -> (20.1046, -94.6736)
  line L790 (19.9148, -94.7519) -> (19.9083, -94.7127)
  line L791 (19.9083, -94.7127) -> (19.8993, -94.674)
  line L792 (19.8387, -94.5276) -> (19.8177, -94.4938)
  line L793 (19.8738, -94.5988) -> (19.8574, -94.5626)
  line L794 (19.7694, -145.5685) -> (19.7946, -145.5378)
  line L795 (19.8177, -94.4938) -> (19.7946, -94.4616)
  line L796 (19.8878, -145.3633) -> (19.8993, -145.3253)
  line L797 (19.7422, -145.5975) -> (19.7694, -145.5685)
  line L798 (19.8574, -145.4367) -> (19.8738, -145.4005)
  line L799 (19.8993, -145.3253) -> (19.9083, -145.2866)
  line L800 (19.8878, -145.3633) -> (19.8993, -145.3253)
  line L801 (20.0587, -94.5222) -> (20.0369, -94.4741)
  line L802 (20.0369, -145.5252) -> (20.0587, -145.4771)
  line L803 (20.1046, -94.6736) -> (20.0926, -94.6222)
  line L804 (19.8738, -145.4005) -> (19.8878, -145.3633)
  line L805 (19.9083, -145.2866) -> (19.9148, -145.2474)
  line L806 (19.92, -94.8997) -> (19.9187, -94.7914)
  line L807 (19.9841, -94.3827) -> (19.9533, -94.3397)
  line L808 (19.8574, -145.4367) -> (19.8738, -145.4005)
  line L809 (19.9187, -94.7914) -> (19.9148, -94.7519)
  line L810 (20.12, -145.1715) -> (20.12, -141.4997)
  line L811 (19.8993, -94.674) -> (19.8878, -94.636)
  line L812 (19.8878, -94.636) -> (19.8738, -94.5988)
  line L813 (19.9533, -94.3397) -> (19.9198, -94.2989)
  line L814 (19.92, -145.1682) -> (19.92, -141.4997)
  line L815 (19.92, -145.1682) -> (19.92, -141.4997)
  line L816 (19.92, -94.8997) -> (19.9187, -94.7914)
  line L817 (20.1184, -145.221) -> (20.12, -145.1715)
  line L818 (19.8387, -94.5276) -> (19.8177, -94.4938)
  line L819 (19.92, -141.4997) -> (19.92, -140.4997)
  line L820 (19.7946, -94.4616) -> (19.7694, -94.4308)
  arc A59 (19.92, -140.4997) -> (19.42, -139.9997) centre (19.42, -140.4997) ccw
  arc A60 (19.92, -140.4997) -> (19.42, -139.9997) centre (19.42, -140.4997) ccw
  line L821 (20.12, -141.4997) -> (20.12, -140.4997)
  line L822 (19.9083, -94.7127) -> (19.8993, -94.674)
  line L823 (19.8574, -94.5626) -> (19.8387, -94.5276)
  line L824 (19.92, -141.4997) -> (19.92, -140.4997)
  line L825 (19.9187, -145.2079) -> (19.92, -145.1682)
  line L826 (19.8738, -94.5988) -> (19.8574, -94.5626)
  line L827 (19.9187, -94.7914) -> (19.9148, -94.7519)
  line L828 (13.82, -150.1995) -> (13.6201, -149.9997)
  line L829 (18.12, -153.2625) -> (18.12, -155.4997)
  line L830 (9.713, -153.8997) -> (9.92, -153.6927)
  line L831 (13.82, -150.1995) -> (13.6201, -149.9997)
  line L832 (19.8859, -154.2627) -> (18.6028, -152.9797)
  line L833 (19.7422, -154.4019) -> (18.4614, -153.1211)
  line L834 (17.92, -153.2625) -> (17.92, -155.2997)
  line L835 (9.713, -153.8997) -> (9.92, -153.6927)
  line L836 (14.02, -109.8826) -> (14.02, -107.2432)
  line L837 (12.7593, -153.8997) -> (16.1593, -157.2997)
  line L838 (13.82, -152.839) -> (13.82, -150.1995)
  line L839 (10.127, -153.8997) -> (12.7593, -153.8997)
  line L840 (16.4807, -155.4997) -> (13.82, -152.839)
  line L841 (16.5635, -155.2997) -> (14.02, -152.7562)
  line L842 (9.92, -153.9755) -> (10.0441, -154.0997)
  line L843 (19.7422, -154.4019) -> (18.4614, -153.1211)
  line L844 (15.42, -138.1997) -> (13.1828, -138.1997)
  line L845 (3.6807, -102.6997) -> (1.72, -102.6997)
  line L846 (15.22, -143.3562) -> (12.6765, -145.8997)
  line L847 (1.72, -102.6997) -> (1.72, -97.2997)
  line L848 (1.92, -102.4997) -> (1.92, -97.4997)
  line L849 (3.2765, -95.2997) -> (1.92, -95.2997)
  line L850 (1.92, -97.4997) -> (3.7635, -97.4997)
  line L851 (1.72, -97.2997) -> (3.6807, -97.2997)
  line L852 (1.72, -102.6997) -> (1.72, -97.2997)
  line L853 (13.82, -147.1603) -> (16.4807, -144.4997)
  line L854 (3.7635, -102.4997) -> (1.92, -102.4997)
  line L855 (13.82, -147.1603) -> (16.4807, -144.4997)
  line L856 (15.42, -138.1997) -> (13.1828, -138.1997)
  line L857 (3.6807, -102.6997) -> (1.72, -102.6997)
  line L858 (3.3593, -95.4997) -> (1.72, -95.4997)
  line L859 (3.3593, -95.4997) -> (1.72, -95.4997)
  line L860 (1.72, -97.2997) -> (3.6807, -97.2997)
  line L861 (14.3222, -140.1775) -> (13.0414, -141.4582)
  line L862 (13.0414, -138.5411) -> (14.3222, -139.8219)
  line L863 (15.22, -137.9997) -> (13.1828, -137.9997)
  line L864 (-0.0459, -105.7366) -> (1.2372, -107.0197)
  line L865 (14.3222, -140.1775) -> (13.0414, -141.4582)
  line L866 (-0.0683, -105.2866) -> (-0.0593, -105.3253)
  line L867 (-0.0683, -105.2866) -> (-0.0593, -105.3253)
  line L868 (13.0414, -138.5411) -> (14.3222, -139.8219)
  line L869 (13.1828, -141.7997) -> (15.42, -141.7997)
  line L870 (14.1831, -139.9656) -> (14.2193, -139.9995)
  line L871 (13.1828, -141.9997) -> (15.22, -141.9997)
  line L872 (15.42, -143.439) -> (12.7593, -146.0997)
  line L873 (14.2193, -139.9999) -> (14.1831, -140.0337)
  line L874 (0.0978, -105.5975) -> (1.3786, -106.8782)
  line L875 (0.0978, -105.5975) -> (1.3786, -106.8782)
  line L876 (13.1828, -141.7997) -> (15.42, -141.7997)
  line L877 (19.9083, -85.2866) -> (19.9148, -85.2474)
  line L878 (5.0918, -140.1997) -> (5.1413, -140.198)
  line L879 (19.8738, -85.4005) -> (19.8878, -85.3633)
  line L880 (5.246, -140.1843) -> (5.2975, -140.1723)
  line L881 (19.9198, -85.7004) -> (19.9533, -85.6596)
  line L882 (19.8859, -85.7366) -> (19.9198, -85.7004)
  line L883 (1.42, -140.1997) -> (5.0918, -140.1997)
  line L884 (20.0587, -85.4771) -> (20.0773, -85.4277)
  line L885 (1.42, -139.9997) -> (5.0886, -139.9997)
  line L886 (19.7946, -85.5378) -> (19.8177, -85.5055)
  line L887 (5.0886, -139.9997) -> (1.42, -139.9997)
  line L888 (19.9148, -85.2474) -> (19.9187, -85.2079)
  line L889 (19.7694, -85.5685) -> (19.7946, -85.5378)
  line L890 (5.2837, -140.0319) -> (5.2457, -140.0203)
  line L891 (19.9148, -85.2474) -> (19.9187, -85.2079)
  line L892 (5.0886, -139.9997) -> (1.42, -139.9997)
  line L893 (19.8177, -85.5055) -> (19.8387, -85.4717)
  line L894 (1.42, -139.9997) -> (5.0886, -139.9997)
  line L895 (19.8177, -85.5055) -> (19.8387, -85.4717)
  line L896 (5.0886, -139.9997) -> (5.1283, -139.9984)
  line L897 (18.4614, -86.8782) -> (19.7422, -85.5975)
  line L898 (5.1283, -140.001) -> (5.0886, -139.9997)
  line L899 (5.0886, -139.9997) -> (5.1283, -139.9984)
  arc A61 (17.92, -86.7368) -> (18.6028, -87.0197) centre (18.32, -86.7368) ccw
  line L900 (19.7422, -85.5975) -> (19.7694, -85.5685)
  line L901 (19.92, -85.1682) -> (19.92, -81.4997)
  line L902 (18.6028, -87.0197) -> (19.8859, -85.7366)
  line L903 (6.7986, -141.4582) -> (5.5178, -140.1775)
  line L904 (19.7422, -85.5975) -> (19.7694, -85.5685)
  line L905 (5.1283, -140.001) -> (5.0886, -139.9997)
  line L906 (20.12, -85.1715) -> (20.12, -81.4997)
  line L907 (6.7986, -141.4582) -> (5.5178, -140.1775)
  arc A62 (18.12, -86.7368) -> (18.4614, -86.8782) centre (18.32, -86.7368) ccw
  line L908 (18.4614, -86.8782) -> (19.7422, -85.5975)
  arc A63 (18.12, -86.7368) -> (18.4614, -86.8782) centre (18.32, -86.7368) ccw
  line L909 (16.4807, -84.4997) -> (18.12, -84.4997)
  line L910 (6.94, -141.3168) -> (5.6569, -140.0337)
  line L911 (16.5635, -84.6997) -> (17.92, -84.6997)
  line L912 (20.1184, -85.221) -> (20.12, -85.1715)
  line L913 (-0.0478, -145.3633) -> (-0.0338, -145.4005)
  line L914 (-0.0683, -145.2866) -> (-0.0593, -145.3253)
  line L915 (0.0013, -145.4717) -> (0.0223, -145.5055)
  line L916 (-0.0748, -145.2474) -> (-0.0683, -145.2866)
  line L917 (16.4807, -84.4997) -> (18.12, -84.4997)
  line L918 (17.92, -84.6997) -> (17.92, -86.7368)
  line L919 (19.92, -85.1682) -> (19.92, -81.4997)
  line L920 (-0.0174, -145.4367) -> (0.0013, -145.4717)
  line L921 (18.12, -84.4997) -> (18.12, -86.7368)
  line L922 (-0.0174, -145.4367) -> (0.0013, -145.4717)
  line L923 (-0.2187, -145.4771) -> (-0.1969, -145.5252)
  line L924 (-0.0748, -145.2474) -> (-0.0683, -145.2866)
  line L925 (18.12, -84.4997) -> (18.12, -86.7368)
  line L926 (0.0706, -145.5685) -> (0.0978, -145.5975)
  line L927 (19.9187, -85.2079) -> (19.92, -85.1682)
  line L928 (-0.0478, -145.3633) -> (-0.0338, -145.4005)
  line L929 (19.9187, -85.2079) -> (19.92, -85.1682)
  line L930 (-0.2646, -145.3257) -> (-0.2526, -145.3771)
  line L931 (-0.1441, -145.6166) -> (-0.1133, -145.6596)
  line L932 (-0.0683, -145.2866) -> (-0.0593, -145.3253)
  line L933 (-0.0798, -145.7004) -> (-0.0459, -145.7366)
  line L934 (0.0223, -145.5055) -> (0.0454, -145.5378)
  line L935 (13.6201, -89.9997) -> (13.82, -89.7998)
  line L936 (-0.0593, -145.3253) -> (-0.0478, -145.3633)
  line L937 (-0.2786, -145.2189) -> (-0.2732, -145.2736)
  line L938 (-0.2732, -145.2736) -> (-0.2646, -145.3257)
  line L939 (0.0223, -145.5055) -> (0.0454, -145.5378)
  line L940 (-0.0593, -145.3253) -> (-0.0478, -145.3633)
  arc A64 (12.9, -81.3168) -> (13.1828, -81.9997) centre (13.1828, -81.5997) ccw
  line L941 (-0.172, -145.5718) -> (-0.1441, -145.6166)
  line L942 (0.0454, -145.5378) -> (0.0706, -145.5685)
  line L943 (-0.1969, -145.5252) -> (-0.172, -145.5718)
  line L944 (-0.1133, -145.6596) -> (-0.0798, -145.7004)
  line L945 (10.127, -86.0997) -> (9.92, -86.3066)
  line L946 (13.82, -90.1995) -> (13.6201, -89.9997)
  line L947 (-0.0787, -145.2079) -> (-0.0748, -145.2474)
  line L948 (-0.2526, -145.3771) -> (-0.2373, -145.4277)
  line L949 (0.0454, -145.5378) -> (0.0706, -145.5685)
  line L950 (-0.0338, -145.4005) -> (-0.0174, -145.4367)
  line L951 (-0.2373, -145.4277) -> (-0.2187, -145.4771)
  line L952 (9.92, -86.0238) -> (9.7959, -85.8997)
  line L953 (9.92, -86.3066) -> (9.713, -86.0997)
  arc A65 (0.42, -139.9997) -> (-0.08, -140.4997) centre (0.42, -140.4997) ccw
  line L954 (0.0013, -145.4717) -> (0.0223, -145.5055)
  line L955 (14.02, -90.1167) -> (13.903, -89.9997)
  arc A66 (13.0414, -81.4582) -> (13.1828, -81.7997) centre (13.1828, -81.5997) ccw
  line L956 (13.1828, -81.9997) -> (15.22, -81.9997)
  line L957 (-0.0338, -145.4005) -> (-0.0174, -145.4367)
  line L958 (-0.08, -140.4997) -> (-0.08, -141.4997)
  line L959 (13.903, -89.9997) -> (14.02, -89.8826)
  line L960 (-0.0787, -145.2079) -> (-0.0748, -145.2474)
  line L961 (14.02, -89.8826) -> (14.02, -87.2432)
  line L962 (13.1828, -81.7997) -> (15.42, -81.7997)
  line L963 (12.6765, -85.8997) -> (10.0441, -85.8997)
  line L964 (15.42, -81.7997) -> (15.42, -83.439)
  line L965 (0.0706, -145.5685) -> (0.0978, -145.5975)
  line L966 (-0.28, -140.4997) -> (-0.28, -141.4997)
  line L967 (13.1828, -81.7997) -> (15.42, -81.7997)
  line L968 (15.22, -83.3562) -> (12.6765, -85.8997)
  line L969 (-0.08, -141.4997) -> (-0.08, -145.0997)
  line L970 (-0.08, -141.4997) -> (-0.08, -145.0997)
  line L971 (10.127, -86.0997) -> (9.92, -86.3066)
  line L972 (13.82, -89.7998) -> (13.82, -87.1603)
  line L973 (15.22, -81.9997) -> (15.22, -83.3562)
  line L974 (9.92, -86.3066) -> (9.713, -86.0997)
  line L975 (-0.0459, -145.7366) -> (1.2372, -147.0197)
  line L976 (0.42, -139.9997) -> (1.42, -139.9997)
  line L977 (15.42, -83.439) -> (12.7593, -86.0997)
  line L978 (-0.28, -145.1009) -> (-0.2786, -145.2189)
  line L979 (1.42, -139.9997) -> (0.42, -139.9997)
  line L980 (10.0441, -85.8997) -> (9.92, -86.0238)
  line L981 (15.42, -83.439) -> (12.7593, -86.0997)
  line L982 (13.82, -87.1603) -> (16.4807, -84.4997)
  line L983 (-0.08, -145.0997) -> (-0.0787, -145.2079)
  line L984 (13.6201, -89.9997) -> (13.82, -89.7998)
  line L985 (1.42, -139.9997) -> (0.42, -139.9997)
  line L986 (12.7593, -86.0997) -> (10.127, -86.0997)
  line L987 (13.82, -89.7998) -> (13.82, -87.1603)
  line L988 (0.42, -139.9997) -> (1.42, -139.9997)
  line L989 (-0.08, -140.4997) -> (-0.08, -141.4997)
  line L990 (15.42, -81.7997) -> (15.42, -83.439)
  line L991 (-0.28, -141.4997) -> (-0.28, -145.1009)
  line L992 (-0.08, -145.0997) -> (-0.0787, -145.2079)
  line L993 (13.82, -90.1995) -> (13.6201, -89.9997)
  line L994 (0.42, -140.1997) -> (1.42, -140.1997)
  arc A67 (13.0414, -81.4582) -> (13.1828, -81.7997) centre (13.1828, -81.5997) ccw
  line L995 (0.0978, -145.5975) -> (1.3786, -146.8782)
  line L996 (12.7593, -86.0997) -> (10.127, -86.0997)
  line L997 (0.0978, -145.5975) -> (1.3786, -146.8782)
  arc A68 (0.42, -139.9997) -> (-0.08, -140.4997) centre (0.42, -140.4997) ccw
  line L998 (14.02, -87.2432) -> (16.5635, -84.6997)
  line L999 (5.82, -87.2432) -> (5.82, -89.8826)
  line L1000 (5.246, -139.8151) -> (5.1939, -139.8065)
  line L1001 (5.1939, -139.8065) -> (5.1413, -139.8013)
  line L1002 (6.6572, -137.9997) -> (4.62, -137.9997)
  line L1003 (5.4888, -139.849) -> (5.5178, -139.8219)
  line L1004 (5.82, -89.8826) -> (5.937, -89.9997)
  line L1005 (5.3974, -139.861) -> (5.348, -139.8424)
  line L1006 (5.2975, -139.8271) -> (5.246, -139.8151)
  line L1007 (6.02, -89.7998) -> (6.2199, -89.9997)
  line L1008 (6.2199, -89.9997) -> (6.02, -90.1995)
  line L1009 (5.4888, -139.849) -> (5.5178, -139.8219)
  line L1010 (13.82, -87.1603) -> (16.4807, -84.4997)
  line L1011 (5.1413, -139.8013) -> (5.0918, -139.7997)
  line L1012 (5.348, -139.8424) -> (5.2975, -139.8271)
  line L1013 (6.02, -87.1603) -> (6.02, -89.7998)
  line L1014 (5.937, -89.9997) -> (5.82, -90.1167)
  arc A69 (6.7986, -138.5411) -> (6.6572, -138.1997) centre (6.6572, -138.3997) ccw
  line L1015 (6.02, -89.7998) -> (6.2199, -89.9997)
  line L1016 (6.6572, -138.1997) -> (4.42, -138.1997)
  line L1017 (6.02, -87.1603) -> (6.02, -89.7998)
  line L1018 (6.6572, -138.1997) -> (4.42, -138.1997)
  line L1019 (19.7422, -105.5975) -> (19.7694, -105.5685)
  line L1020 (19.7422, -105.5975) -> (19.7694, -105.5685)
  line L1021 (19.8993, -105.3253) -> (19.9083, -105.2866)
  line L1022 (18.4614, -106.8782) -> (19.7422, -105.5975)
  line L1023 (19.8387, -105.4717) -> (19.8574, -105.4367)
  line L1024 (19.8738, -105.4005) -> (19.8878, -105.3633)
  line L1025 (19.8177, -105.5055) -> (19.8387, -105.4717)
  arc A70 (18.12, -106.7368) -> (18.4614, -106.8782) centre (18.32, -106.7368) ccw
  arc A71 (17.92, -106.7368) -> (18.6028, -107.0197) centre (18.32, -106.7368) ccw
  line L1026 (18.12, -104.4997) -> (18.12, -106.7368)
  line L1027 (17.92, -104.6997) -> (17.92, -106.7368)
  line L1028 (18.12, -104.4997) -> (18.12, -106.7368)
  line L1029 (18.4614, -106.8782) -> (19.7422, -105.5975)
  arc A72 (18.12, -106.7368) -> (18.4614, -106.8782) centre (18.32, -106.7368) ccw
  line L1030 (20.0773, -105.4277) -> (20.0926, -105.3771)
  line L1031 (5.82, -152.7562) -> (3.2765, -155.2997)
  line L1032 (6.02, -152.839) -> (3.3593, -155.4997)
  line L1033 (1.3786, -153.1211) -> (0.0978, -154.4019)
  line L1034 (19.8859, -105.7366) -> (19.9198, -105.7004)
  line L1035 (7.1635, -154.0997) -> (9.7959, -154.0997)
  line L1036 (1.72, -155.4997) -> (1.72, -153.2625)
  line L1037 (19.8993, -105.3253) -> (19.9083, -105.2866)
  line L1038 (3.7635, -157.4997) -> (7.1635, -154.0997)
  line L1039 (19.7946, -105.5378) -> (19.8177, -105.5055)
  line L1040 (19.8574, -105.4367) -> (19.8738, -105.4005)
  line L1041 (7.0807, -153.8997) -> (9.713, -153.8997)
  line L1042 (1.3786, -153.1211) -> (0.0978, -154.4019)
  line L1043 (19.9083, -105.2866) -> (19.9148, -105.2474)
  line L1044 (7.0807, -153.8997) -> (9.713, -153.8997)
  line L1045 (19.8738, -105.4005) -> (19.8878, -105.3633)
  line L1046 (19.9187, -105.2079) -> (19.92, -105.0997)
  line L1047 (19.7694, -105.5685) -> (19.7946, -105.5378)
  line L1048 (19.7694, -105.5685) -> (19.7946, -105.5378)
  line L1049 (3.6807, -157.2997) -> (7.0807, -153.8997)
  line L1050 (1.2372, -152.9797) -> (-0.0459, -154.2627)
  line L1051 (3.6807, -157.2997) -> (7.0807, -153.8997)
  line L1052 (20.1132, -105.2736) -> (20.1186, -105.2189)
  line L1053 (1.92, -155.2997) -> (1.92, -153.2625)
  line L1054 (20.0369, -105.5252) -> (20.0587, -105.4771)
  line L1055 (20.0926, -105.3771) -> (20.1046, -105.3257)
  line L1056 (19.92, -154.8997) -> (19.9187, -154.7914)
  line L1057 (19.8993, -154.674) -> (19.8878, -154.636)
  line L1058 (19.8574, -154.5626) -> (19.8387, -154.5276)
  line L1059 (20.0926, -154.6222) -> (20.0773, -154.5717)
  line L1060 (19.8878, -154.636) -> (19.8738, -154.5988)
  line L1061 (19.8878, -154.636) -> (19.8738, -154.5988)
  line L1062 (19.8387, -154.5276) -> (19.8177, -154.4938)
  line L1063 (20.12, -154.8985) -> (20.1186, -154.7804)
  line L1064 (19.7946, -154.4616) -> (19.7694, -154.4308)
  line L1065 (3.2765, -195.2997) -> (1.92, -195.2997)
  line L1066 (14.5425, -220.1723) -> (14.594, -220.1843)
  line L1067 (-0.0787, -45.2079) -> (-0.0748, -45.2474)
  line L1068 (-0.2187, -45.4771) -> (-0.1969, -45.5252)
  line L1069 (14.5943, -219.979) -> (14.633, -219.988)
  line L1070 (3.3593, -215.4997) -> (1.72, -215.4997)
  arc A73 (1.92, -213.2625) -> (1.2372, -212.9797) centre (1.52, -213.2625) ccw
  line L1071 (-0.2373, -45.4277) -> (-0.2187, -45.4771)
  line L1072 (3.6807, -37.2997) -> (7.0807, -33.8997)
  line L1073 (1.3786, -193.1211) -> (0.0978, -194.4019)
  line L1074 (-0.2732, -45.2736) -> (-0.2646, -45.3257)
  line L1075 (1.3786, -193.1211) -> (0.0978, -194.4019)
  line L1076 (-0.0748, -45.2474) -> (-0.0683, -45.2866)
  line L1077 (14.3945, -220.1165) -> (14.4426, -220.1383)
  line L1078 (18.12, -182.6997) -> (16.1593, -182.6997)
  line L1079 (14.5191, -219.9534) -> (14.5563, -219.9674)
  line L1080 (1.92, -35.2997) -> (1.92, -33.2625)
  line L1081 (-0.0478, -45.3633) -> (-0.0338, -45.4005)
  line L1082 (-0.0338, -45.4005) -> (-0.0174, -45.4367)
  line L1083 (3.3593, -195.4997) -> (1.72, -195.4997)
  line L1084 (14.4479, -219.9183) -> (14.483, -219.9371)
  line L1085 (14.5563, -219.9674) -> (14.5943, -219.979)
  line L1086 (14.7117, -219.9984) -> (14.7514, -219.9997)
  line L1087 (14.3512, -219.849) -> (14.3819, -219.8742)
  line L1088 (17.92, -177.4997) -> (17.92, -182.4997)
  line L1089 (6.02, -212.839) -> (3.3593, -215.4997)
  line L1090 (18.12, -182.6997) -> (16.1593, -182.6997)
  arc A74 (1.72, -213.2625) -> (1.3786, -213.1211) centre (1.52, -213.2625) ccw
  line L1091 (14.3819, -219.8742) -> (14.4142, -219.8974)
  line L1092 (0.0013, -45.4717) -> (0.0223, -45.5055)
  line L1093 (-0.1969, -34.4741) -> (-0.2187, -34.5222)
  line L1094 (3.3593, -215.4997) -> (1.72, -215.4997)
  line L1095 (14.2601, -220.033) -> (14.303, -220.0637)
  line L1096 (-0.0338, -45.4005) -> (-0.0174, -45.4367)
  line L1097 (1.72, -215.4997) -> (1.72, -213.2625)
  line L1098 (14.5191, -219.9534) -> (14.5563, -219.9674)
  line L1099 (16.1593, -177.2997) -> (18.12, -177.2997)
  line L1100 (14.3479, -220.0916) -> (14.3945, -220.1165)
  line L1101 (0.0223, -45.5055) -> (0.0454, -45.5378)
  line L1102 (14.5943, -219.979) -> (14.633, -219.988)
  line L1103 (14.303, -220.0637) -> (14.3479, -220.0916)
  line L1104 (-0.1969, -45.5252) -> (-0.172, -45.5718)
  line L1105 (-0.0683, -45.2866) -> (-0.0593, -45.3253)
  line L1106 (-0.1441, -45.6166) -> (-0.1133, -45.6596)
  arc A75 (1.72, -213.2625) -> (1.3786, -213.1211) centre (1.52, -213.2625) ccw
  line L1107 (1.72, -195.4997) -> (1.72, -193.2625)
  line L1108 (0.0223, -45.5055) -> (0.0454, -45.5378)
  line L1109 (-0.0593, -45.3253) -> (-0.0478, -45.3633)
  arc A76 (1.92, -193.2625) -> (1.2372, -192.9797) centre (1.52, -193.2625) ccw
  line L1110 (1.72, -195.4997) -> (1.72, -193.2625)
  line L1111 (1.92, -195.2997) -> (1.92, -193.2625)
  line L1112 (1.72, -215.4997) -> (1.72, -213.2625)
  line L1113 (17.92, -182.4997) -> (16.0765, -182.4997)
  line L1114 (-0.0593, -45.3253) -> (-0.0478, -45.3633)
  line L1115 (18.12, -177.2997) -> (18.12, -182.6997)
  line L1116 (1.92, -215.2997) -> (1.92, -213.2625)
  line L1117 (18.12, -177.2997) -> (18.12, -182.6997)
  line L1118 (14.6461, -220.1929) -> (14.6987, -220.198)
  line L1119 (-0.08, -45.0997) -> (-0.0787, -45.2079)
  line L1120 (14.5563, -219.9674) -> (14.5943, -219.979)
  line L1121 (14.633, -219.988) -> (14.6722, -219.9945)
  line L1122 (16.0765, -177.4997) -> (17.92, -177.4997)
  line L1123 (3.2765, -215.2997) -> (1.92, -215.2997)
  line L1124 (0.0706, -45.5685) -> (0.0978, -45.5975)
  line L1125 (14.492, -220.1569) -> (14.5425, -220.1723)
  line L1126 (-0.172, -194.4275) -> (-0.1969, -194.4741)
  line L1127 (-0.2526, -45.3771) -> (-0.2373, -45.4277)
  line L1128 (-0.2646, -45.3257) -> (-0.2526, -45.3771)
  line L1129 (14.4426, -220.1383) -> (14.492, -220.1569)
  line L1130 (-0.0174, -194.5626) -> (-0.0338, -194.5988)
  line L1131 (16.1593, -177.2997) -> (18.12, -177.2997)
  line L1132 (-0.0593, -194.674) -> (-0.0683, -194.7127)
  line L1133 (14.7514, -219.9997) -> (18.42, -219.9997)